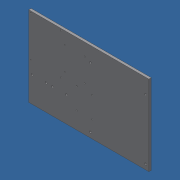
# Autodesk Inventor part: BackPlate
Saved by Autodesk Inventor 2021 (Build 250183000, 183)
## iProperties
Created: 2022-08-30
Part Number: BackPlate
Material: Generic
Document SubType Name: Modeling
Designer: Nathann
Density: 1 g/cm^3
Appearance: Default
Author: Nathann
Autodesk Inventor part; units mm, degrees
ref_plane "YZ Plane" through (0, 0, 0) normal (1, 0, 0) x (0, 1, 0)
ref_plane "XZ Plane" through (0, 0, 0) normal (0, 1, 0) x (-1, 0, 0)
ref_plane "XY Plane" through (0, 0, 0) normal (0, 0, 1) x (1, 0, 0)
sketch "Sketch1" plane through (0, 0, 0) normal (0, 1, 0) x (-1, 0, 0)
  line L0 (-150, -100) -> (150, -100)
  line L1 (150, -100) -> (150, 100)
  line L2 (150, 100) -> (-150, 100)
  line L3 (-150, 100) -> (-150, -100)
  line L4 (-150, -100) -> (150, 100) construction
  line L5 (150, -100) -> (-150, 100) construction
  point P0 (0, 0)
  dimension "d2" = 200
  dimension "d3" = 300
  constraints: 12 end point, 2 midpoint, 2 parallel, 1 horizontal, 1 perpendicular
  measures "d2" distance of L2.end L0.start
  measures "d3" distance of L0.start L0.end
extrude "Extrusion1" add sketch "Sketch1" along normal blind 6
sketch "Sketch2" plane through (0, 0, 0) normal (0, -1, 0) x (1, 0, 0)
  ellipse E0 centre (142.032, -87.3608) end of major axis (142.032, -84.8608) minor radius 2.5 projected
  ellipse E1 centre (142.0329, 62.6392) end of major axis (142.0329, 60.1392) minor radius 2.5 projected
  ellipse E2 centre (4.033, 62.6392) end of major axis (4.033, 60.1392) minor radius 2.5 projected
  ellipse E3 centre (4.0321, -87.3608) end of major axis (4.0321, -84.8608) minor radius 2.5 projected
  ellipse E4 centre (-55.6025, -36.4196) end of major axis (-55.6025, -38.9196) minor radius 2.5 projected
  ellipse E5 centre (-90.6023, -36.5399) end of major axis (-90.6023, -39.0399) minor radius 2.5 projected
  ellipse E6 centre (-106.647, -36.3461) end of major axis (-106.647, -38.8461) minor radius 2.5 projected
  ellipse E7 centre (-141.6465, -36.5286) end of major axis (-141.6465, -39.0286) minor radius 2.5 projected
  ellipse E8 centre (-30.4377, -58.095) end of major axis (-30.4377, -59.695) minor radius 1.6 projected
  ellipse E9 centre (8.5622, -58.1864) end of major axis (8.5622, -59.7864) minor radius 1.6 projected
  ellipse E10 centre (8.6864, -5.1866) end of major axis (8.6864, -6.7866) minor radius 1.6 projected
  ellipse E11 centre (-30.3134, -5.0951) end of major axis (-30.3134, -6.6951) minor radius 1.6 projected
  ellipse E12 centre (-59.3931, 10.7278) end of major axis (-59.3931, 12.0778) minor radius 1.35 projected
  ellipse E13 centre (-10.3932, 10.6651) end of major axis (-10.3932, 12.0151) minor radius 1.35 projected
  ellipse E14 centre (-10.3189, 68.665) end of major axis (-10.3189, 70.015) minor radius 1.35 projected
  ellipse E15 centre (-59.3188, 68.7278) end of major axis (-59.3188, 70.0778) minor radius 1.35 projected
  ellipse E16 centre (-68.9752, 95.6258) end of major axis (-68.9751, 93.8758) minor radius 1.7487 projected
  ellipse E17 centre (-68.9684, -6.3742) end of major axis (-68.9683, -8.1242) minor radius 1.7487 projected
  ellipse E18 centre (-144.911, -6.3793) end of major axis (-144.9109, -8.1293) minor radius 1.7487 projected
  ellipse E19 centre (-144.9178, 95.6207) end of major axis (-144.9177, 93.8707) minor radius 1.7487 projected
  point P0 (0, 0)
  point P1 (-95.5494, -69.6074)
  point P2 (-98.0151, -68.8063)
  constraints: 9 other
extrude "Extrusion2" cut sketch "Sketch2" against normal mid plane 30
equation "\"RodDiameter\" = 8"
equation "\"VerticalBearingOD\" = 16"
equation "\"PrintingClearance\" = 0.2"
equation "\"TubeID\" = 18"
body "Solid1"
